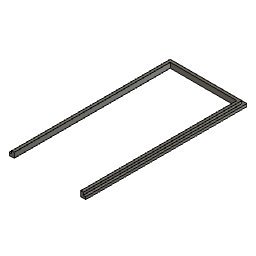
DoorFrame (Autodesk Fusion 360 design; units mm, degrees)
Autodesk Fusion 360 part; units mm, degrees
sketch "Sketch1" plane through (0, 0, 0) normal (0, 1, 0) x (1, 0, 0)
  line L0 (0, 0) -> (15, 0)
  line L1 (15, 0) -> (15, 31.5)
  line L2 (15, 31.5) -> (0, 31.5)
  line L3 (0, 31.5) -> (0, 0)
  line L4 (1, 0) -> (14, 0)
  line L5 (14, 0) -> (14, 30.5)
  line L6 (14, 30.5) -> (1, 30.5)
  line L7 (1, 30.5) -> (1, 0)
  line L8 (0.5, 0) -> (14.5, 0)
  line L9 (14.5, 0) -> (14.5, 31)
  line L10 (14.5, 31) -> (0.5, 31)
  line L11 (0.5, 31) -> (0.5, 0)
  dimension "d1" = 15
  dimension "d2" = 31.5
  dimension "d3" = 13
  dimension "d4" = 30.5
  dimension "d5" = 1
  dimension "d6" = 14
  dimension "d7" = 31
  dimension "d8" = 0.5
  constraint horizontal L0
  constraint vertical L1
  constraint horizontal L2
  constraint vertical L3
  constraint coincident L0.start L3.end
  constraint horizontal L4
  constraint vertical L5
  constraint horizontal L6
  constraint vertical L7
  constraint coincident L0 L4.start
  constraint horizontal L8
  constraint vertical L9
  constraint horizontal L10
  constraint vertical L11
  constraint coincident L0 L8.start
  measures "d1" distance of L0.start L0.end
  measures "d2" distance of L0.start L2.end
  measures "d3" distance of L4.start L4.end
  measures "d4" distance of L4.start L6.end
  measures "d5" distance of L1 L5
  measures "d6" distance of L8.start L8.end
  measures "d7" distance of L8.start L10.end
  measures "d8" distance of L1 L9
extrude "Extrude1" add sketch "Sketch1" along normal blind 0.5 contours L0 L1 L2 L3 L9 L10 L11
extrude "Extrude2" add sketch "Sketch1" along normal blind 1 contours L0 L5 L6 L7 L8 L9 L10 L11
